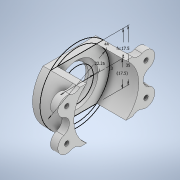
# Autodesk Inventor part: shaft holder
Saved by Autodesk Inventor 2020.3 (Build 243373000, 373)
## iProperties
Created: 2020-08-09
Part Number: shaft holder
Material: Generic
Document SubType Name: Modeling
Designer: joesp
Density: 1 g/cm^3
Appearance: Default
Author: joesp
Autodesk Inventor part; units mm, degrees
ref_plane "YZ Plane" through (0, 0, 0) normal (1, 0, 0) x (0, 1, 0)
ref_plane "XZ Plane" through (0, 0, 0) normal (0, 1, 0) x (-1, 0, 0)
ref_plane "XY Plane" through (0, 0, 0) normal (0, 0, 1) x (1, 0, 0)
sketch "Sketch1" plane through (0, 0, 0) normal (1, 0, 0) x (0, 1, 0)
  circle A0 centre (0, 0) radius 11.125
  line L0 (17.5, 17.8536) -> (17.5, -17.8536)
  line L1 (-17.5, 17.8536) -> (-17.5, -17.8536)
  circle A1 centre (0, 0) radius 25
  circle A2 centre (0, 0) radius 22
  point P0 (-17.5, -13.3323)
  point P1 (17.5, -13.3323)
  point P2 (17.5, 13.3323)
  point P3 (-17.5, 13.3323)
  dimension "d0" = 22.25
  dimension "d1" = 44
  dimension "d2" = 3
  dimension "d3" = 35
  dimension "d4" = 17.5
  dimension "d5" = 17.5
  constraints: 4 end point, 4 point on circle, 3 centre point, 3 coincident, 2 vertical
  measures "d0" diameter of A0
  measures "d1" diameter of A2
  measures "d2" radial gap between concentric circles of A1 A2
  measures "d3" distance between parallel lines of L1 L0
  measures "d4" distance from line of point (0, 0) L0
  measures "d5" distance from line of point (0, 0) L1
extrude "Extrusion1" add sketch "Sketch1" against normal blind 5 contours L0 A2 L1
sketch "Sketch2" plane through (0, 0, 0) normal (0, 1, 0) x (-1, 0, 0)
  circle A0 centre (1, -12.125) radius 2.5
  line L0 (0, -11.125) -> (0, 11.125) projected
  line L1 (0, -13.3323) -> (5, -13.3323) projected
  line L2 (10.1054, 0) -> (-6.8503, 0) construction
  point P0 (0, 0)
  dimension "d8" = 5
  dimension "d9" = 1
  dimension "d11" = 1
  constraints: 2 end point, 1 centre point, 1 coincident, 1 horizontal
  measures "d8" diameter of A0
  measures "d9" distance from line of L0 A0.centre
  measures "d11" horizontal distance of point (0, -11.125) A0.centre
revolve "Revolution1" cut sketch "Sketch2" angle 360 about axis through (-10.1054, 0, 0) along (1, 0, 0)
extrude "Extrusion2" add sketch "Sketch1" along normal blind 20 and the other way blind 5 contours L0 A2 L1 A1 | L0 A1 L1 A2
sketch "Sketch3" plane through (20, 0, 0) normal (1, 0, 0) x (0, 0, -1)
  line L0 (-13.3323, 17.5) -> (-17.8536, 17.5) projected
  arc A0 (-24.2536, 16.374) -> (-17.8536, 17.5) centre (-21.8402, 21.4076) ccw
  arc A1 (-24.2536, 16.374) -> (-28.7823, 5.2842) centre (-26.8477, 10.9637) ccw
  arc A2 (-17.8536, 17.5) -> (-17.8536, -17.5) centre (0, 0) ccw projected
  arc A3 (-25, 0) -> (-28.7823, 5.2842) centre (-30.5823, 0) ccw
  arc A4 (-28.7823, -5.2842) -> (-25, 0) centre (-30.5823, 0) ccw
  arc A5 (-28.7823, -5.2842) -> (-24.2536, -16.374) centre (-26.8477, -10.9637) ccw
  arc A6 (-17.8536, -17.5) -> (-24.2536, -16.374) centre (-21.8402, -21.4076) ccw
  arc A7 (-17.8536, 17.5) -> (-17.8536, -17.5) centre (0, 0) ccw projected
  line L1 (-17.8536, 17.5) -> (17.8536, 17.5) projected
  arc A8 (17.8536, 17.5) -> (24.2536, 16.374) centre (21.8402, 21.4076) ccw
  arc A9 (28.7823, 5.2842) -> (24.2536, 16.374) centre (26.8477, 10.9637) ccw
  arc A10 (28.7823, 5.2842) -> (25, 0) centre (30.5823, 0) ccw
  line L2 (17.8536, -17.5) -> (-17.8536, -17.5) projected
  arc A11 (24.2536, -16.374) -> (17.8536, -17.5) centre (21.8402, -21.4076) ccw
  arc A12 (24.2536, -16.374) -> (28.7823, -5.2842) centre (26.8477, -10.9637) ccw
  arc A13 (25, 0) -> (28.7823, -5.2842) centre (30.5823, 0) ccw
  arc A14 (17.8536, -17.5) -> (17.8536, 17.5) centre (0, 0) ccw projected
  circle A15 centre (-26.8477, -10.9637) radius 4 construction
  circle A16 centre (-26.8477, 10.9637) radius 4 construction
  circle A17 centre (26.8477, 10.9637) radius 4 construction
  circle A18 centre (26.8477, -10.9637) radius 4 construction
  dimension "d17" = 6
  dimension "d18" = 6
  dimension "d19" = 6
  dimension "d20" = 6
  dimension "d21" = 8
  dimension "d22" = 8
  dimension "d23" = 8
  dimension "d24" = 8
  constraints: 27 point on circle, 19 tangent, 16 centre point, 4 coincident, 2 equal radius, 2 horizontal alignment, 2 vertical alignment
  measures "d17" radius of A5
  measures "d18" radius of A12
  measures "d19" radius of A1
  measures "d20" radius of A9
  measures "d21" diameter of A15
  measures "d22" diameter of A16
  measures "d23" diameter of A17
  measures "d24" diameter of A18
extrude "Extrusion3" add sketch "Sketch3" against normal blind 5 contours A2 A3 A1 A0 | A8 A9 A10 A14 | A2 A6 A5 A4 | A13 A12 A11 A14
sketch "Sketch4" plane through (15, 0, 0) normal (-1, 0, 0) x (0, 0, 1)
  line L0 (22.2714, -11.5895) -> (24.0176, -7.3135)
  line L1 (24.0176, -7.3135) -> (28.5938, -6.6877)
  line L2 (28.5938, -6.6877) -> (31.4239, -10.3379)
  line L3 (31.4239, -10.3379) -> (29.6777, -14.6139)
  line L4 (29.6777, -14.6139) -> (25.1015, -15.2397)
  line L5 (25.1015, -15.2397) -> (22.2714, -11.5895)
  line L6 (25.1015, 15.2397) -> (29.6777, 14.6139)
  line L7 (29.6777, 14.6139) -> (31.4239, 10.3379)
  line L8 (31.4239, 10.3379) -> (28.5938, 6.6877)
  line L9 (28.5938, 6.6877) -> (24.0176, 7.3135)
  line L10 (24.0176, 7.3135) -> (22.2714, 11.5895)
  line L11 (22.2714, 11.5895) -> (25.1015, 15.2397)
  line L12 (-25.1015, -15.2397) -> (-29.6777, -14.6139)
  line L13 (-29.6777, -14.6139) -> (-31.4239, -10.3379)
  line L14 (-31.4239, -10.3379) -> (-28.5938, -6.6877)
  line L15 (-28.5938, -6.6877) -> (-24.0176, -7.3135)
  line L16 (-24.0176, -7.3135) -> (-22.2714, -11.5895)
  line L17 (-22.2714, -11.5895) -> (-25.1015, -15.2397)
  line L18 (-29.6777, 14.6139) -> (-25.1015, 15.2397)
  line L19 (-25.1015, 15.2397) -> (-22.2714, 11.5895)
  line L20 (-22.2714, 11.5895) -> (-24.0176, 7.3135)
  line L21 (-24.0176, 7.3135) -> (-28.5938, 6.6877)
  line L22 (-28.5938, 6.6877) -> (-31.4239, 10.3379)
  line L23 (-31.4239, 10.3379) -> (-29.6777, 14.6139)
  arc A0 (17.8536, -17.5) -> (17.8536, 17.5) centre (0, 0) ccw projected
  arc A1 (-17.8536, 17.5) -> (-17.8536, -17.5) centre (0, 0) ccw projected
  arc A2 (24.2536, -16.374) -> (17.8536, -17.5) centre (21.8402, -21.4076) ccw projected
  arc A3 (25, 0) -> (28.7823, -5.2842) centre (30.5823, 0) ccw projected
  arc A4 (28.7823, 5.2842) -> (25, 0) centre (30.5823, 0) ccw projected
  arc A5 (17.8536, 17.5) -> (24.2536, 16.374) centre (21.8402, 21.4076) ccw projected
  arc A6 (-17.8536, -17.5) -> (-24.2536, -16.374) centre (-21.8402, -21.4076) ccw projected
  arc A7 (-28.7823, -5.2842) -> (-25, 0) centre (-30.5823, 0) ccw projected
  arc A8 (-25, 0) -> (-28.7823, 5.2842) centre (-30.5823, 0) ccw projected
  arc A9 (-24.2536, 16.374) -> (-17.8536, 17.5) centre (-21.8402, 21.4076) ccw projected
  point P0 (26.8477, -10.9637)
  point P1 (26.8477, 10.9637)
  point P2 (-26.8477, -10.9637)
  point P3 (-26.8477, 10.9637)
  point P4 (23.1445, 9.4515)
  point P5 (23.1445, -9.4515)
  point P6 (-23.1445, -9.4515)
  point P7 (-23.1445, 9.4515)
  dimension "d27" = 8
  dimension "d30" = 8
  dimension "d31" = 8
  dimension "d32" = 8
  dimension "d33" = 11.5823
  dimension "d34" = 11.5823
  dimension "d35" = 11.5823
  dimension "d36" = 11.5823
  dimension "d37" = 11.5823
  dimension "d38" = 11.5823
  dimension "d39" = 11.5823
  dimension "d40" = 11.5823
  constraints: 48 end point, 4 midpoint, 4 point on circle, 4 tangent, 52 other
  measures "d27" distance between parallel lines of L10 L7
  measures "d30" distance between parallel lines of L0 L3
  measures "d31" distance between parallel lines of L13 L16
  measures "d32" distance between parallel lines of L23 L20
  measures "d33" distance of A2.centre point (26.848, -10.964)
  measures "d34" distance of A3.centre point (26.848, -10.964)
  measures "d35" distance of A4.centre point (26.848, 10.964)
  measures "d36" distance of A5.centre point (26.848, 10.964)
  measures "d37" distance of A6.centre point (-26.848, -10.964)
  measures "d38" distance of A7.centre point (-26.848, -10.964)
  measures "d39" distance of A8.centre point (-26.848, 10.964)
  measures "d40" distance of A9.centre point (-26.848, 10.964)
extrude "Extrusion4" cut sketch "Sketch4" against normal blind 2.5
sketch "Sketch5" plane through (17.5, 0, 0) normal (-1, 0, 0) x (0, 0, 1)
  circle A0 centre (-26.8477, -10.9637) radius 1.5
  circle A1 centre (-26.8477, 10.9637) radius 1.5
  circle A2 centre (26.8477, 10.9637) radius 1.5
  circle A3 centre (26.8477, -10.9637) radius 1.5
  line L0 (29.6777, -14.6139) -> (25.1015, -15.2397) projected
  line L1 (24.0176, -7.3135) -> (28.5938, -6.6877) projected
  line L2 (31.4239, -10.3379) -> (29.6777, -14.6139) projected
  line L3 (23.1445, -9.4515) -> (24.0176, -7.3135) projected
  line L4 (28.5938, 6.6877) -> (24.0176, 7.3135) projected
  line L5 (25.1015, 15.2397) -> (29.6777, 14.6139) projected
  line L6 (23.1445, 9.4515) -> (22.2714, 11.5895) projected
  line L7 (29.6777, 14.6139) -> (31.4239, 10.3379) projected
  line L8 (-28.5938, 6.6877) -> (-31.4239, 10.3379) projected
  line L9 (-25.1015, 15.2397) -> (-22.2714, 11.5895) projected
  line L10 (-24.0176, 7.3135) -> (-28.5938, 6.6877) projected
  line L11 (-29.6777, 14.6139) -> (-25.1015, 15.2397) projected
  line L12 (-25.1015, -15.2397) -> (-29.6777, -14.6139) projected
  line L13 (-28.5938, -6.6877) -> (-24.0176, -7.3135) projected
  line L14 (-31.4239, -10.3379) -> (-28.5938, -6.6877) projected
  line L15 (-22.2714, -11.5895) -> (-25.1015, -15.2397) projected
  point P0 (0, 0)
  dimension "d43" = 4
  dimension "d44" = 4
  dimension "d45" = 4
  dimension "d46" = 4
  dimension "d47" = 3
  dimension "d48" = 3
  dimension "d49" = 4
  dimension "d50" = 4
  dimension "d51" = 4
  dimension "d52" = 4
  dimension "d53" = 3
  dimension "d54" = 3
  dimension "d55" = 4
  dimension "d56" = 4
  dimension "d57" = 4
  dimension "d58" = 4
  dimension "d59" = 4
  dimension "d60" = 4
  dimension "d61" = 4
  dimension "d62" = 4
  constraints: 4 centre point
  measures "d43" distance from line of L0 A3.centre
  measures "d44" distance from line of L1 A3.centre
  measures "d45" distance from line of L2 A3.centre
  measures "d46" distance from line of L3 A3.centre
  measures "d47" diameter of A3
  measures "d48" diameter of A2
  measures "d49" distance from line of L4 A2.centre
  measures "d50" distance from line of L5 A2.centre
  measures "d51" distance from line of L6 A2.centre
  measures "d52" distance from line of L7 A2.centre
  measures "d53" diameter of A1
  measures "d54" diameter of A0
  measures "d55" distance from line of L8 A1.centre
  measures "d56" distance from line of L9 A1.centre
  measures "d57" distance from line of L10 A1.centre
  measures "d58" distance from line of L11 A1.centre
  measures "d59" distance from line of L12 A0.centre
  measures "d60" distance from line of L13 A0.centre
  measures "d61" distance from line of L14 A0.centre
  measures "d62" distance from line of L15 A0.centre
extrude "Extrusion5" cut sketch "Sketch5" against normal through all
equation "\"d4\" = d5"
equation "\"d18\" = d17"
equation "\"d19\" = d17"
equation "\"d20\" = d17"
equation "\"d22\" = d21"
equation "\"d23\" = d21"
equation "\"d24\" = d21"
equation "\"d33\" = d34"
equation "\"d35\" = d36"
equation "\"d37\" = d38"
equation "\"d39\" = d40"
equation "\"d43\" = d44"
equation "\"d45\" = d46"
equation "\"d49\" = d50"
equation "\"d51\" = d52"
equation "\"d55\" = d56"
equation "\"d57\" = d58"
equation "\"d59\" = d60"
equation "\"d61\" = d62"
body "Solid1"
